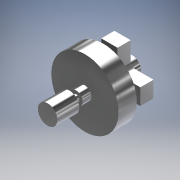
# Autodesk Inventor part: BrImp_Motormodel
Saved by Autodesk Inventor 2018 (Build 220112000, 112)
## iProperties
Created: 2018-02-04
Part Number: BrImp_Motormodel
Material: Aluminum 6061
Document SubType Name: Modeling
Designer: Benedikt
Density: 2.7 g/cm^3
Appearance: Aluminum - Flat
Author: Benedikt
Autodesk Inventor part; units mm, degrees
ref_plane "YZ Plane" through (0, 0, 0) normal (1, 0, 0) x (0, 1, 0)
ref_plane "XZ Plane" through (0, 0, 0) normal (0, 1, 0) x (-1, 0, 0)
ref_plane "XY Plane" through (0, 0, 0) normal (0, 0, 1) x (1, 0, 0)
sketch "Sketch1" plane through (0, 0, 0) normal (0, 1, 0) x (-1, 0, 0)
  circle A0 centre (0, 0) radius 15.3
  dimension "d0" = 30.6
  constraints: 1 centre point, 1 coincident
  measures "d0" diameter of A0
extrude "Extrusion1" add sketch "Sketch1" against normal blind 8.35
sketch "Sketch2" plane through (0, 0, 0) normal (0, 1, 0) x (1, 0, 0)
  circle A0 centre (0, 0) radius 4
  dimension "d3" = 8
  constraints: 1 centre point, 1 coincident
  measures "d3" diameter of A0
extrude "Extrusion2" add sketch "Sketch2" along normal blind 2.8
sketch "Sketch3" plane through (0, 2.8, 0) normal (0, 1, 0) x (1, 0, 0)
  line L0 (-3.7, 14.1) -> (3.7, 14.1)
  line L1 (3.7, -14.1) -> (-3.7, -14.1)
  line L2 (-3.7, 14.1) -> (3.7, -14.1) construction
  line L3 (3.7, 14.1) -> (-3.7, -14.1) construction
  line L4 (14.1, 3.7) -> (14.1, -3.7)
  line L5 (-14.1, -3.7) -> (-14.1, 3.7)
  line L6 (-14.1, 3.7) -> (14.1, -3.7) construction
  line L7 (14.1, 3.7) -> (-14.1, -3.7) construction
  line L8 (3.7, 14.1) -> (3.7, 5.2221)
  line L9 (3.7, -5.2221) -> (3.7, -14.1)
  line L10 (14.1, -3.7) -> (5.2221, -3.7)
  line L11 (-5.2221, -3.7) -> (-14.1, -3.7)
  line L12 (-14.1, 3.7) -> (-5.2221, 3.7)
  line L13 (5.2221, 3.7) -> (14.1, 3.7)
  line L14 (-3.7, -14.1) -> (-3.7, -5.2221)
  line L15 (-3.7, 5.2221) -> (-3.7, 14.1)
  arc A0 (3.7, -5.2221) -> (5.2221, -3.7) centre (0, 0) ccw
  arc A1 (-5.2221, -3.7) -> (-3.7, -5.2221) centre (0, 0) ccw
  arc A2 (5.2221, 3.7) -> (3.7, 5.2221) centre (0, 0) ccw
  arc A3 (-3.7, 5.2221) -> (-5.2221, 3.7) centre (0, 0) ccw
  dimension "d6" = 7.4
  dimension "d7" = 28.2
  dimension "d8" = 28.2
  dimension "d9" = 7.4
  constraints: 32 end point, 10 parallel, 8 point on circle, 4 centre point, 4 midpoint, 4 perpendicular, 3 horizontal, 1 coincident
  measures "d6" distance of L1.start L1.end
  measures "d7" distance of L0.end L1.start
  measures "d8" distance of L4.end L5.start
  measures "d9" distance of L4.start L4.end
extrude "Extrusion3" add sketch "Sketch3" along normal blind 6
sketch "Sketch4" plane through (0, 8.8, 0) normal (0, 1, 0) x (1, 0, 0)
  circle A0 centre (0, 0) radius 4
  dimension "d13" = 8
  constraints: 1 centre point, 1 coincident
  measures "d13" diameter of A0
extrude "Extrusion4" add sketch "Sketch4" along normal blind 4.5
sketch "Sketch5" plane through (0, -8.35, 0) normal (0, -1, 0) x (1, 0, 0)
  circle A0 centre (0, 0) radius 4 projected
  circle A1 centre (0, 0) radius 3
  dimension "d16" = 6
  constraints: 1 centre point, 1 coincident
  measures "d16" diameter of A1
extrude "Extrusion5" add sketch "Sketch5" along normal blind 4 contours A1
sketch "Sketch6" plane through (0, -12.35, 0) normal (0, -1, 0) x (1, 0, 0)
  circle A0 centre (0, 0) radius 1.5
  dimension "d19" = 3
  constraints: 1 centre point, 1 coincident
  measures "d19" diameter of A0
extrude "Extrusion6" add sketch "Sketch6" along normal blind 13
sketch "Sketch7" plane through (0, -25.35, 0) normal (0, -1, 0) x (1, 0, 0)
  circle A0 centre (0, 0) radius 4.45
  dimension "d22" = 8.9
  constraints: 1 centre point, 1 coincident
  measures "d22" diameter of A0
extrude "Extrusion7" add sketch "Sketch7" against normal blind 10
body "Solid1"
